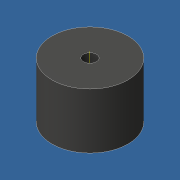
# Autodesk Inventor part: GummiFeet
Saved by Autodesk Inventor 2016 (Build 200138000, 138)
## iProperties
Created: 2016-02-29
Part Number: GummiFeet
Material: Gummi, Silikon
Document SubType Name: Modeling
Designer: 4ndreas
Density: 1.25 g/cm^3
Appearance: Gummi - schwarz
Mass: 33.3948 g
Surface Area: 60.5119 cm^2
Volume: 26.7158 cm^3
Author: 4ndreas
Autodesk Inventor part; units mm, degrees
ref_plane "YZ Plane" through (0, 0, 0) normal (1, 0, 0) x (0, 1, 0)
ref_plane "XZ Plane" through (0, 0, 0) normal (0, 1, 0) x (-1, 0, 0)
ref_plane "XY Plane" through (0, 0, 0) normal (0, 0, 1) x (1, 0, 0)
sketch "Skizze1" plane through (0, 0, 0) normal (0, 0, 1) x (1, 0, 0)
  circle A0 centre (0, 0) radius 18.5
  dimension "d0" = 37
  constraints: 1 centre point, 1 coincident
  measures "d0" diameter of A0
extrude "Extrusion1" add sketch "Skizze1" along normal blind 27
sketch "Skizze2" plane through (0, 0, 0) normal (0, 0, -1) x (-1, 0, 0)
  circle A0 centre (0, 0) radius 7
  dimension "d3" = 14
  constraints: 1 centre point, 1 coincident
  measures "d3" diameter of A0
extrude "Extrusion2" cut sketch "Skizze2" against normal blind 12
sketch "Skizze3" plane through (0, 0, 12) normal (0, 0, -1) x (-1, 0, 0)
  point P0 (0, 0)
hole "Bohrung1" at (0, 0, 12) direction (0, 0, 1) diameter 6.3 end through all
